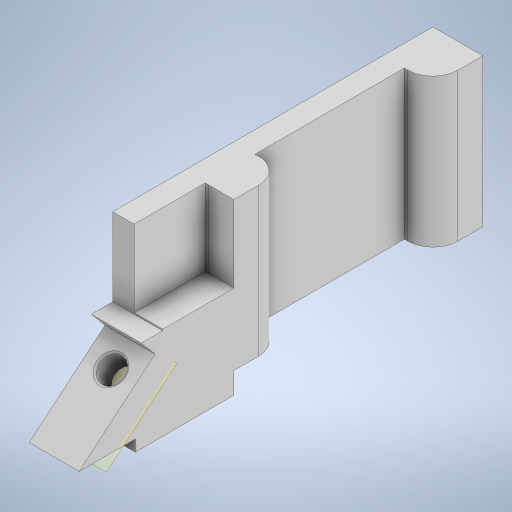
# Autodesk Inventor part: ściana
Saved by Autodesk Inventor 2023 (Build 270158000, 158)
## iProperties
Created: 2025-01-11
Part Number: ściana
Material: Ogólny
Document SubType Name: Modeling
Designer: kamil
Density: 1 g/cm^3
Appearance: Domyślna
Author: kamil
Autodesk Inventor part; units mm, degrees
ref_plane "YZ Plane" through (0, 0, 0) normal (1, 0, 0) x (0, 1, 0)
ref_plane "XZ Plane" through (0, 0, 0) normal (0, 1, 0) x (-1, 0, 0)
ref_plane "XY Plane" through (0, 0, 0) normal (0, 0, 1) x (1, 0, 0)
sketch "Szkic1" plane through (0, 0, 0) normal (1, 0, 0) x (0, 1, 0)
  line L0 (0, 0) -> (10, 0)
  line L1 (10, 0) -> (10, -55)
  line L2 (10, -55) -> (0, -55)
  line L3 (0, -55) -> (0, 0)
  dimension "d0" = 10
  dimension "d1" = 55
  constraints: 8 end point, 2 parallel, 1 horizontal, 1 perpendicular
  measures "d0" distance of L1.end L2.end
  measures "d1" distance of L0.end L1.end
extrude "Wyciągnięcie proste1" add sketch "Szkic1" along normal blind 7
sketch "Szkic2" plane through (0, 0, 0) normal (-1, 0, 0) x (0, 0, 1)
  line L0 (7.3328, -6.25) -> (12, -6.25) projected
  line L1 (12, -6.25) -> (-7.1511, 9.8197) projected
  line L2 (-7.1511, 9.8197) -> (-9.0795, 7.5216) projected
  line L3 (7.3328, -6.25) -> (-9.0795, 7.5216) projected
  line L4 (-55, 0) -> (-55, 10) projected
  line L5 (0, 0) -> (-55, 0) projected
  line L6 (0, 10) -> (0, 0) projected
  line L7 (-55, 10) -> (0, 10) projected
  line L8 (-7.1511, 9.8197) -> (-7.1511, 12.4768)
  point P0 (-7.1511, 10)
  point P1 (-0.1156, 0)
  constraints: 2 end point, 1 vertical
extrude "Wyciągnięcie proste2" cut sketch "Szkic2" against normal blind 10 contours L3 L2 L1 L6 L5 | L1 L8 L7 L6
sketch "Szkic3" plane through (0, 7.5216, -9.0795) normal (0, 0.7660444, 0.6427876) x (1, 0, 0)
  circle A0 centre (3.5, -3.5) radius 1.6 projected
  point P0 (0, -11.79)
hole "Otwór1" at (3.5, 5.2718, -6.3983) direction (0, -0.7660444, -0.6427876) diameter 3.5 end through all countersink diameter 4 countersink angle 90
ref_plane "Płaszczyzna konstrukcyjna1" through (0, 4.8404, -11.3292) normal (0, 0.7660444, 0.6427876) x (1, 0, 0)
sketch "Szkic5" plane through (0, 0, 0) normal (-1, 0, 0) x (0, 0, 1)
  line L0 (-0.1156, 0) -> (-9.0795, 7.5216) projected
  line L1 (-9.0795, 7.5216) -> (-7.1511, 9.8197) projected
  line L2 (-7.1511, 9.8197) -> (-7.1511, 10) projected
  line L3 (-55, 10) -> (-7.1511, 10) projected
  line L4 (-55, 0) -> (-55, 10) projected
  line L5 (-0.1156, 0) -> (-55, 0) projected
  line L6 (-0.1156, 0) -> (3.4596, -3)
  line L7 (-20.1156, 0) -> (-20.1156, -3)
  line L8 (-20.1156, -3) -> (3.4596, -3)
  point P0 (0, 0)
  dimension "d17" = 20
  dimension "d18" = 3
  dimension "d19" = 40
  constraints: 6 end point, 1 horizontal, 1 point on line, 1 vertical
  measures "d17" distance of L7.start L0.start
  measures "d18" distance between parallel lines of L8 L5
  measures "d19" angle of L8 L6
extrude "Wyciągnięcie proste4" add sketch "Szkic5" against normal up to surface (7 mm away) contours L6 L8 L7 L5
sketch "Szkic4" plane through (0, 4.8404, -11.3292) normal (0, 0.7660444, 0.6427876) x (1, 0, 0)
  circle A0 centre (3.5, -3.5) radius 1.75 projected
  circle A1 centre (3.5, -3.5) radius 2.9
  line L0 (6.4, -5.1743) -> (3.5, -6.8486)
  line L1 (3.5, -6.8486) -> (0.6, -5.1743)
  line L2 (0.6, -5.1743) -> (0.6, -1.8257)
  line L3 (0.6, -1.8257) -> (3.5, -0.1514)
  line L4 (3.5, -0.1514) -> (6.4, -1.8257)
  line L5 (6.4, -1.8257) -> (6.4, -5.1743)
  point P0 (0, -11.79)
  point P1 (6.4, -3.5)
  dimension "d14" = 5.8
  constraints: 12 end point, 2 coincident, 1 horizontal alignment, 1 midpoint, 15 other
extrude "Wyciągnięcie proste3" cut sketch "Szkic4" against normal through all contours A0 | A1 | L5 L0 A1 | A1 L4 L5 | A1 L3 L4 | L0 L1 A1 | A1 L2 L3 | L1 L2 A1
sketch "Szkic6" plane through (0, 0, 0) normal (-1, 0, 0) x (0, 0, 1)
  line L0 (-6.0829, 0.4382) -> (-8.9679, -3) projected
  line L1 (-6.0829, 0.4382) -> (-3.602, 3.3948)
  line L2 (3.4596, -3) -> (-9.0795, 7.5216) projected
  line L3 (4.2983, -3) -> (-6.3199, -3)
  line L4 (-6.3199, -3) -> (-6.3199, -1.4)
  line L5 (-6.3199, -1.4) -> (4.2983, -1.4)
  line L6 (4.2983, -1.4) -> (4.2983, -3)
  line L7 (-20.1156, -3) -> (3.4596, -3) projected
  line L8 (-8.899, -4.4737) -> (-6.014, -1.0355)
  line L9 (-6.014, -1.0355) -> (-2.8359, 2.752)
  point P0 (0, 0)
  point P1 (1.5528, -1.4)
  dimension "d22" = 1.6
  dimension "d23" = 1
  constraints: 14 end point, 2 parallel, 1 collinear, 1 horizontal, 1 perpendicular, 1 point on line, 1 other
  measures "d22" distance of L3.end L4.end
  measures "d23" distance between parallel lines of L0 L8
extrude "Wyciągnięcie proste5" cut sketch "Szkic6" against normal through all contours L4 L5 L2 L3
sketch "Szkic7" plane through (0, 10, -55) normal (0, 1, 0) x (1, 0, 0)
  line L0 (0, -47.8489) -> (7, -47.8489) projected
  line L1 (7, 0) -> (7, -47.8489) projected
  line L2 (0, 0) -> (7, 0) projected
  line L3 (0, 0) -> (0, -47.8489) projected
  circle A0 centre (3.5, -3.5) radius 3.5
  line L4 (0, -34.8844) -> (7, -34.8844) projected
  circle A1 centre (3.5, -31.3844) radius 3.5
  line L5 (3, -27.8844) -> (7, -27.8844)
  line L6 (7, -27.8844) -> (7, -7)
  line L7 (7, -7) -> (3, -7)
  line L8 (3, -7) -> (3, -27.8844)
  point P0 (0, -55)
  point P1 (3.5, 0)
  point P2 (7, -3.5)
  point P3 (3.5, -7)
  point P4 (3.5, -27.8844)
  point P5 (7, -31.3844)
  dimension "d26" = 7
  dimension "d27" = 3.5
  dimension "d28" = 7
  dimension "d29" = 3.5
  dimension "d30" = 4
  constraints: 8 end point, 2 centre point, 2 parallel, 2 tangent, 2 vertical alignment, 1 horizontal, 1 midpoint, 1 perpendicular, 1 point on line
  measures "d26" diameter of A0
  measures "d27" distance from line of A0.centre L2
  measures "d28" diameter of A1
  measures "d29" distance from line of L4 A1.centre
  measures "d30" distance between parallel lines of L1 L8
extrude "Wyciągnięcie proste6" cut sketch "Szkic7" against normal through all contours A1 L5 L1 | L5 L8 L7 L1 | A0 L1 L7
sketch "Szkic9" plane through (0, 10, -55) normal (0, 1, 0) x (1, 0, 0)
  arc A0 (7, -31.3844) -> (3.5, -27.8844) centre (3.5, -31.3844) ccw projected
  line L0 (3.5, -27.8844) -> (3, -27.8844) projected
  line L1 (3, -27.8844) -> (3, -7) projected
  line L2 (3, -7) -> (3.5, -7) projected
  arc A1 (3.5, -7) -> (7, -3.5) centre (3.5, -3.5) ccw projected
  line L3 (7, 0) -> (7, -3.5) projected
  line L4 (0, 0) -> (7, 0) projected
  line L5 (0, 0) -> (0, -47.8489) projected
  line L6 (0, -47.8489) -> (7, -47.8489) projected
  line L7 (7, -31.3844) -> (7, -47.8489) projected
  line L8 (3, -7) -> (3, 0)
  line L9 (3, -27.8844) -> (3, -47.8489)
  point P0 (0, -55)
  constraints: 4 end point, 3 point on line, 1 vertical
extrude "Wyciągnięcie proste7" add sketch "Szkic9" along normal blind 10.75 contours L9 L6 L5 L4 L8 L1
sketch "Szkic10" plane through (0, 9.8197, -7.1511) normal (0, 0, 1) x (1, 0, 0)
  line L0 (7, 0.1803) -> (7, 0) projected
  line L1 (3, 0.1803) -> (7, 0.1803) projected
  line L2 (3, 0.1803) -> (3, 10.9303) projected
  line L3 (0, 10.9303) -> (3, 10.9303) projected
  line L4 (0, 0) -> (0, 10.9303) projected
  line L5 (0, 0) -> (7, 0) projected
  line L6 (0, -9.8197) -> (0, 10.9303) projected
  line L7 (0, 10.9303) -> (7, 10.9303)
  line L8 (7, 10.9303) -> (7, 0.1803)
  line L9 (7, 0.1803) -> (0, 0.1803)
  line L10 (0, 0.1803) -> (0, 10.9303)
  constraints: 8 end point, 2 parallel, 1 horizontal, 1 perpendicular
extrude "Wyciągnięcie proste8" cut sketch "Szkic10" against normal blind 3 contours L0 L5 L4 L9 L1 | L9 L4 L3 L2
sketch "Szkic11" plane through (3, 10, -55) normal (0, 1, 0) x (1, 0, 0)
  line L0 (0, 0) -> (0, -7) projected
  line L1 (0, -7) -> (0.5, -7) projected
  arc A0 (0.5, -7) -> (4, -3.5) centre (0.5, -3.5) ccw projected
  line L2 (4, 0) -> (4, -3.5) projected
  line L3 (0, 0) -> (4, 0) projected
  line L4 (0, -44.8489) -> (4, -44.8489) projected
  line L5 (4, -31.3844) -> (4, -44.8489) projected
  arc A1 (4, -31.3844) -> (0.5, -27.8844) centre (0.5, -31.3844) ccw projected
  line L6 (0.5, -27.8844) -> (0, -27.8844) projected
  line L7 (0, -27.8844) -> (0, -44.8489) projected
  circle A2 centre (0.5, -31.3844) radius 3.5
  line L8 (4, -34.8844) -> (-3, -34.8844) projected
  line L9 (0.5, -34.8844) -> (4, -34.8844)
  line L10 (4, -34.8844) -> (4, -31.3844)
  line L11 (4, -31.3844) -> (0.5, -31.3844)
  line L12 (0.5, -31.3844) -> (0.5, -34.8844)
  line L13 (-3, -34.8844) -> (-3, -48.6801) projected
  line L14 (0.5, -31.3844) -> (-3, -31.3844)
  line L15 (-3, -31.3844) -> (-3, -34.8844)
  line L16 (-3, -34.8844) -> (0.5, -34.8844)
  line L17 (0.5, -34.8844) -> (0.5, -31.3844)
  point P0 (-3, -55)
  point P1 (0.5, -34.8844)
  constraints: 16 end point, 4 parallel, 2 horizontal, 2 perpendicular, 1 coincident, 1 midpoint, 1 point on line, 4 other
extrude "Wyciągnięcie proste9" add sketch "Szkic11" along normal up to surface (10.75 mm away) contours L3 L2 A0 L1 L0 | L8 A2 L5 | A2 L14 L7 | L7 L14 L12 A2 | L12 L11 A2 | L11 L14 L7 A2 A1 | L14 A2 L7
